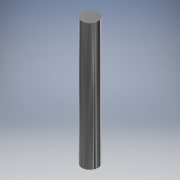
# Autodesk Inventor part: guia_linear_12mm_150mm
Saved by Autodesk Inventor 2018 (Build 220112000, 112)
## iProperties
Created: 2018-05-10
Part Number: guia_linear_12mm_150mm
Material: Aço inoxidável
Document SubType Name: Modelagem
Designer: Georgines
Density: 8 g/cm^3
Appearance: Semipolido
Sheet Metal Rule: Padrão
Mass: 81.2944 g
Surface Area: 36.1591 cm^2
Volume: 10.1618 cm^3
Author: Georgines
Autodesk Inventor part; units mm, degrees
ref_plane "YZ Plane" through (0, 0, 0) normal (1, 0, 0) x (0, 1, 0)
ref_plane "XZ Plane" through (0, 0, 0) normal (0, 1, 0) x (-1, 0, 0)
ref_plane "XY Plane" through (0, 0, 0) normal (0, 0, 1) x (1, 0, 0)
sketch "Esboço1" plane through (0, 0, 0) normal (0, 0, 1) x (1, 0, 0)
  circle A0 centre (0, 0) radius 5.995
  dimension "d0" = 11.99
  constraints: 1 centre point, 1 coincident
  measures "d0" diameter of A0
extrude "Extrusão1" add sketch "Esboço1" along normal mid plane 94.76
equation "\"Raio_vergadura\" = Espessura"
equation "\"Largura_alívio_de_vergadura\" = Espessura"
equation "\"Profundidade_alívio_de_vergadura\" = 0.5 * Espessura"
equation "\"Tamanho_alívio_de_dobra\" = 4 * Espessura"
equation "\"Remanescente_mínimo\" = 2 * Espessura"
equation "\"Raiodetransição\" = Raio_vergadura"
equation "\"Tamanho_de_raio_de_Jacobi\" = Espessura"
equation "\"TamanhoFolga\" = Espessura"
equation "\"Espessura\" = 0.5"
